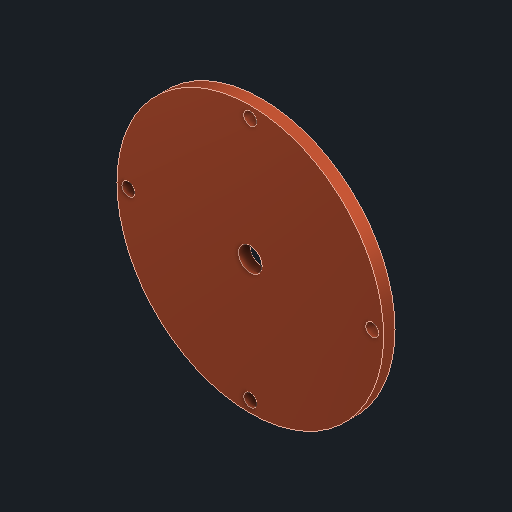
# Autodesk Inventor part: anode_holder
Saved by Autodesk Inventor 2025 (Build 290162000, 162)
## iProperties
Created: 2024-05-20
Part Number: anode_holder
Material: Copper
Document SubType Name: Modeling
Designer: queezz
Density: 8.94 g/cm^3
Appearance: Copper - Satin
Author: queezz
Autodesk Inventor part; units mm, degrees
ref_plane "YZ Plane" through (0, 0, 0) normal (1, 0, 0) x (0, 1, 0)
ref_plane "XZ Plane" through (0, 0, 0) normal (0, 1, 0) x (-1, 0, 0)
ref_plane "XY Plane" through (0, 0, 0) normal (0, 0, 1) x (1, 0, 0)
sketch "Sketch1" plane through (0, 0, 0) normal (0, 0, 1) x (1, 0, 0)
  circle A0 centre (0, 0) radius 35
  dimension "d0" = 70
  constraints: 1 centre point, 1 coincident
  measures "d0" diameter of A0
extrude "Extrusion1" add sketch "Sketch1" along normal blind 3
sketch "Sketch2" plane through (0, 0, 3) normal (0, 0, 1) x (1, 0, 0)
  circle A0 centre (0, 0) radius 32 construction
  point P0 (32, 0)
  dimension "d3" = 64
  constraints: 2 horizontal alignment, 1 coincident, 2 other
hole "Hole1" at (32, 0, 3) direction (0, 0, -1) diameter 3.4 depth 10 tip angle 118
pattern_circular "Circular Pattern1" count 4 over 360 about axis through (0, 0, 0) along (0, 0, 1) of "Hole1"
hole "Hole2" at (0, 0, 0) direction (0, 0, 1) diameter 6.2 end through all
body "Solid1"
